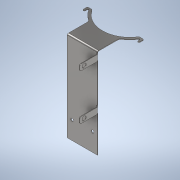
# Autodesk Inventor part: Glass fixer plate
Saved by Autodesk Inventor 2020.3 (Build 243373000, 373)
## iProperties
Created: 2020-06-30
Part Number: Glass fixer plate
Material: Steel, Carbon
Document SubType Name: Sheet Metal
Designer: Bruno
Density: 7.85 g/cm^3
Sheet Metal Rule: Default_mm
Appearance: Semi-Polished
Author: Bruno
Autodesk Inventor part; units mm, degrees
ref_plane "YZ Plane" through (0, 0, 0) normal (1, 0, 0) x (0, 1, 0)
ref_plane "XZ Plane" through (0, 0, 0) normal (0, 1, 0) x (-1, 0, 0)
ref_plane "XY Plane" through (0, 0, 0) normal (0, 0, 1) x (1, 0, 0)
sketch "Sketch1" plane through (0, 0, 0) normal (0, 0, 1) x (1, 0, 0)
  line L0 (0, 0) -> (50, 0)
  line L1 (50, 0) -> (50, 150)
  line L2 (50, 150) -> (0, 150)
  line L3 (0, 150) -> (0, 0)
  dimension "d0" = 50
  dimension "d1" = 150
  measures "d0" distance of L2.end L1.end
  measures "d1" distance of L1.end L0.end
extrude "Plate1" add sketch "Sketch1" along normal blind 1
sketch "Sketch2" plane through (50, 149, 1) normal (0, 1, 0) x (-1, 0, 0)
  line L0 (50, 0) -> (0, 0)
  line L1 (0, 0) -> (0, -79)
  line L2 (0, -79) -> (50, -79)
  line L3 (50, -79) -> (50, 0)
  constraints: 6 end point, 1 horizontal, 1 perpendicular, 1 vertical
edge flange "Flange1" height 79 angle 90 thickness 1 bend radius 1 thickness toward (0, 1, 0) relief straight relief width 1 relief depth 0.5 edges at (25, 150, 0) wall of the first edge with corners at (0, 149, 1) (50, 149, 1) (50, 149, -78) (0, 149, -78)
bend "Bend1"
corner "Corner1"
sketch "Sketch4" plane through (0, 150, -78) normal (0, 1, 0) x (1, 0, 0)
  line L0 (0, 0) -> (50, 0)
  line L1 (0, 0) -> (-40, 0)
  line L2 (-40, 0) -> (-40, -40)
  line L3 (-40, -40) -> (0, -40)
  line L4 (0, -40) -> (0, 0)
  line L5 (50, -77) -> (50, 0)
  line L6 (50, 0) -> (90, 0)
  line L7 (90, 0) -> (90, -40)
  line L8 (90, -40) -> (50, -40)
  line L9 (50, -40) -> (50, 0)
  point P0 (0, -78)
  dimension "d14" = 40
  dimension "d15" = 40
  dimension "d16" = 40
  dimension "d17" = 40
  measures "d14" distance of L3.end L2.end
  measures "d15" distance of L2.end L1.end
  measures "d16" distance of L7.end L8.end
  measures "d17" distance of L6.end L7.end
sheet face with bend "Face2" sketch "Sketch4" thickness 1 toward (0, -1, 0) bend radius 1 relief straight relief width 1 relief depth 0.5
bend "Bend2"
fillet "Corner Round7" radius 6 2 edges at (0, 149.5, -38) (50, 149.5, -38)
sketch "Sketch3" plane through (0, 150, -78) normal (0, 1, 0) x (1, 0, 0)
  line L0 (0, 0) -> (50, 0) projected
  circle A0 centre (25, 0) radius 45.5
  arc A1 (-16.7744, -26.5) -> (66.7744, -26.5) centre (25, 0) ccw
  arc A2 (0, -46) -> (-6, -40) centre (-6, -46) ccw projected
  circle A3 centre (-6, -46) radius 6
  arc A4 (56, -40) -> (50, -46) centre (56, -46) ccw projected
  circle A5 centre (56, -46) radius 6
  line L1 (-40, -40) -> (-6, -40) projected
  line L2 (-6, -40) -> (-40, -40)
  line L3 (-40, 0) -> (-40, -40) projected
  line L4 (-40, -40) -> (-40, 0)
  line L5 (-40, 0) -> (-20.5, 0)
  line L6 (90, 0) -> (-40, 0) projected
  line L7 (56, -40) -> (90, -40) projected
  line L8 (56, -40) -> (90, -40)
  line L9 (90, -40) -> (90, 0) projected
  line L10 (90, -40) -> (90, 0)
  line L11 (90, 0) -> (70.5, 0)
  line L12 (25, 0) -> (25, -45.5)
  line L13 (25, -45.5) -> (25, -23.5) construction
  line L14 (25, -23.5) -> (63.9615, -23.5) construction
  line L15 (63.9615, -23.5) -> (69.9615, -23.5)
  line L16 (63.9615, -23.5) -> (69.9615, -23.5) construction
  line L17 (71.9615, -25.5) -> (71.9615, -30)
  line L18 (70.4615, -31.5) -> (70.4615, -31.5)
  line L19 (25, -23.5) -> (-13.9615, -23.5) construction
  line L20 (-13.9615, -23.5) -> (-19.9615, -23.5)
  line L21 (-13.9615, -23.5) -> (-7.9615, -23.5) construction
  line L22 (-21.9615, -25.5) -> (-21.9615, -30)
  line L23 (-20.4615, -31.5) -> (-20.4615, -31.5)
  arc A6 (-16.7744, -26.5) -> (66.7744, -26.5) centre (25, 0) ccw
  line L24 (-18.9615, -30) -> (-18.9615, -27.5)
  line L25 (-17.9615, -26.5) -> (-16.7744, -26.5)
  line L26 (68.9615, -30) -> (68.9615, -27.5)
  line L27 (67.9615, -26.5) -> (66.7744, -26.5)
  arc A7 (-19.9615, -23.5) -> (-21.9615, -25.5) centre (-19.9615, -25.5) ccw
  arc A8 (-21.9615, -30) -> (-20.4615, -31.5) centre (-20.4615, -30) ccw
  arc A9 (-20.4615, -31.5) -> (-18.9615, -30) centre (-20.4615, -30) ccw
  arc A10 (-17.9615, -26.5) -> (-18.9615, -27.5) centre (-17.9615, -27.5) ccw
  arc A11 (71.9615, -25.5) -> (69.9615, -23.5) centre (69.9615, -25.5) ccw
  arc A12 (70.4615, -31.5) -> (71.9615, -30) centre (70.4615, -30) ccw
  arc A13 (68.9615, -30) -> (70.4615, -31.5) centre (70.4615, -30) ccw
  arc A14 (68.9615, -27.5) -> (67.9615, -26.5) centre (67.9615, -27.5) ccw
  point P0 (0, -78)
  point P1 (52.6469, -41.0244)
  point P2 (-2.6469, -41.0244)
  point P3 (71.9615, -23.5)
  point P4 (71.9615, -31.5)
  point P5 (68.9615, -31.5)
  point P6 (-21.9615, -23.5)
  point P7 (-21.9615, -31.5)
  point P8 (-18.9615, -31.5)
  point P9 (-18.9615, -26.5)
  point P10 (68.9615, -26.5)
  point P11 (-2.6469, -41.0244)
  point P12 (52.6469, -41.0244)
  point P13 (70.4615, -31.5)
  dimension "d13" = 91
  dimension "d84" = 22
  dimension "d85" = 8
  dimension "d86" = 0
  dimension "d87" = 8
  dimension "d88" = 3
  dimension "d89" = 8
  dimension "d90" = 180
  dimension "d91" = 8
  dimension "d92" = 90
  dimension "d93" = 3
  dimension "d95" = 5
  dimension "d96" = 5
  dimension "d97" = 2
  dimension "d98" = 1.5
  dimension "d99" = 1.5
  dimension "d100" = 1
  dimension "d101" = 2
  dimension "d102" = 1.5
  dimension "d103" = 1
  constraints: 44 end point, 25 point on circle, 19 point on line, 18 tangent, 13 centre point, 7 perpendicular, 6 collinear, 5 horizontal, 4 coincident, 3 vertical, 1 concentric, 1 midpoint
  measures "d13" diameter of A0
  measures "d84" distance of L12.end L13.end
  measures "d85" distance of L14.end point (71.962, -23.5)
  measures "d86" distance between parallel lines of L15 L16
  measures "d87" distance of point (71.962, -23.5) point (71.962, -31.5)
  measures "d88" distance of point (71.962, -31.5) point (68.962, -31.5)
  measures "d89" distance of L19.end point (-21.962, -23.5)
  measures "d90" angle of L20 L21
  measures "d91" distance of point (-21.962, -23.5) point (-21.962, -31.5)
  measures "d92" angle of L22 L20
  measures "d93" distance of point (-21.962, -31.5) point (-18.962, -31.5)
  measures "d95" distance of point (-18.962, -31.5) point (-18.962, -26.5)
  measures "d96" distance of point (68.962, -31.5) point (68.962, -26.5)
  measures "d97" radius of A7
  measures "d98" radius of A8
  measures "d99" radius of A9
  measures "d100" radius of A10
  measures "d101" radius of A11
  measures "d102" radius of A12
  measures "d103" radius of A14
extrude "Extrusion1" cut sketch "Sketch3" against normal through all contours L6 A0 L0 | L0 L12 A0 L6 | L0 L6 A0 L12 | A0 L20 A7 L22 A8 A9 L24 A10 L25 A1 A2 L1 L3 L5 | L6 L9 L7 A4 A1 L27 A14 L26 A13 A12 L17 A11 L15 A0
sketch "Sketch5" plane through (0, 150, -1) normal (0, 1, 0) x (1, 0, 0)
  arc A0 (-13.9615, 53.5) -> (63.9615, 53.5) centre (25, 77) ccw projected
  point P0 (0, -1)
  point P1 (70.5, 77)
  point P2 (-20.5, 77)
sketch "Sketch7" plane through (0, 0, 1) normal (0, 0, 1) x (1, 0, 0)
  line L0 (50, 0) -> (0, 0) projected
  line L1 (0, 0) -> (0, 148) projected
  line L2 (50, 148) -> (50, 0) projected
  point P0 (8, 30)
  point P1 (42, 30)
  dimension "d37" = 30
  dimension "d38" = 8
  dimension "d39" = 8
  constraints: 1 horizontal alignment
  measures "d37" distance from line of L0 point (8, 30)
  measures "d38" distance from line of L1 point (8, 30)
  measures "d39" distance from line of L2 point (42, 30)
hole "Hole1" at (8, 30, 1) at (42, 30, 1) direction (0, 0, -1) diameter 4.5 end through all
fillet "Corner Round12" radius 1 1 edges at (-16.7744, 149.5, -51.5)
fillet "Corner Round13" radius 1 1 edges at (66.7744, 149.5, -51.5)
fillet "Corner Round14" radius 3 1 edges at (63.9615, 149.5, -54.5)
fillet "Corner Round15" radius 3 1 edges at (-13.9615, 149.5, -54.5)
sketch "Sketch10" plane through (0, 150, -1) normal (0, 1, 0) x (1, 0, 0)
  arc A0 (70.7921, 70.1608) -> (-20.7921, 70.1608) centre (25, 77) ccw
  line L0 (25, 77) -> (25, 30.7) construction
  line L1 (-17.3207, 50.5) -> (-17.9615, 50.5) projected
  line L2 (-18.9615, 47) -> (-18.9615, 49.5) projected
  line L3 (-17.6615, 49.2) -> (-20.7921, 70.1608)
  line L4 (-20.7921, 70.1608) -> (25, 70.1608) construction
  line L5 (68.9615, 49.5) -> (68.9615, 47) projected
  line L6 (67.3207, 50.5) -> (67.9615, 50.5) projected
  line L7 (67.6615, 49.2) -> (70.7921, 70.1608)
  line L8 (70.7921, 70.1608) -> (25, 70.1608) construction
  point P0 (0, -1)
  dimension "d109" = 92.6
  dimension "d115" = 1.3
  dimension "d116" = 1.3
  dimension "d117" = 45.7921
  dimension "d118" = 6.8392
  dimension "d119" = 1.3
  dimension "d120" = 1.3
  dimension "d121" = 45.7921
  constraints: 10 end point, 2 point on circle, 2 tangent, 1 centre point, 1 coincident, 1 perpendicular, 1 point on line, 1 vertical
  measures "d109" diameter of A0
  measures "d115" distance from line of L2 L3.start
  measures "d116" distance from line of L1 L3.start
  measures "d117" distance of L3.end L4.end
  measures "d118" distance from line of point (25, 77) L4
  measures "d119" distance from line of L5 L7.start
  measures "d120" distance from line of L7.start L6
  measures "d121" distance of L7.end L4.end
sketch "Sketch13" plane through (50, 0, 0) normal (1, 0, 0) x (0, 0, -1)
  line L0 (-1, 0) -> (-1, 148)
  line L1 (-1, 146) -> (-31, 146)
  line L2 (-31, 146) -> (-31, 136)
  line L3 (-31, 136) -> (-1, 136)
  line L4 (-1, 136) -> (-1, 146)
  line L5 (-1, 70) -> (-31, 70)
  line L6 (-31, 70) -> (-31, 60)
  line L7 (-31, 60) -> (-1, 60)
  line L8 (-1, 60) -> (-1, 70)
  point P0 (0, 0)
  dimension "d133" = 30
  dimension "d134" = 10
  dimension "d135" = 146
  dimension "d136" = 30
  dimension "d137" = 10
  dimension "d138" = 66
  measures "d133" distance of L3.end L2.end
  measures "d134" distance of L2.end L1.end
  measures "d135" distance from line of L0.start L1
  measures "d136" distance of L7.end L6.end
  measures "d137" distance of L6.end L5.end
  measures "d138" distance between parallel lines of L5 L3
sheet face with bend "Face4" sketch "Sketch13" thickness 1 toward (1, 0, 0) bend radius 1 relief straight relief width 1 relief depth 0.5
bend "Bend4"
sketch "Sketch14" plane through (50, 0, 0) normal (-1, 0, 0) x (0, 0, 1)
  line L0 (1, 0) -> (1, 148) projected
  line L1 (2, 146) -> (31, 146) projected
  line L2 (2, 70) -> (31, 70) projected
  point P0 (0, 0)
  point P1 (24, 141)
  point P2 (24, 65)
  dimension "d144" = 23
  dimension "d145" = 5
  dimension "d146" = 5
  dimension "d154" = 76
  constraints: 1 vertical alignment
  measures "d144" distance from line of L0 point (24, 141)
  measures "d145" distance from line of L1 point (24, 141)
  measures "d146" distance from line of point (24, 65) L2
  measures "d154" distance of point (24, 65) point (24, 141)
hole "Hole2" at (50, 141, 24) at (50, 65, 24) direction (1, 0, 0) diameter 7 end through all
fillet "Fillet1" radius 2 4 edges at (50.5, 146, 31) (50.5, 136, 31) (50.5, 70, 31) (50.5, 60, 31)
equation "\"d39\" = d38"
equation "\"d145\" = 0.5 * d134"
equation "\"d146\" = d145"
equation "\"d16\" = d14"
equation "\"d17\" = d15"
equation "\"d45\" = Thickness"
equation "\"d137\" = d134"
equation "\"d152\" = Thickness"
equation "\"d2\" = Thickness"
equation "\"d3\" = BendReliefWidth"
equation "\"d4\" = BendReliefDepth"
equation "\"d5\" = MinimumRemnant"
equation "\"d6\" = TransitionRadius"
equation "\"d9\" = BendRadius"
equation "\"d10\" = CornerReliefSize"
equation "\"d11\" = GapSize"
equation "\"d12\" = JacobiRadiusSize"
equation "\"d18\" = BendRadius"
equation "\"d19\" = BendReliefWidth"
equation "\"d21\" = MinimumRemnant"
equation "\"d20\" = BendReliefDepth"
equation "\"d22\" = TransitionRadius"
equation "\"d139\" = BendRadius"
equation "\"d140\" = BendReliefWidth"
equation "\"d142\" = MinimumRemnant"
equation "\"d141\" = BendReliefDepth"
equation "\"d143\" = TransitionRadius"
equation "\"BendRadius\" = Thickness"
equation "\"BendReliefWidth\" = Thickness"
equation "\"BendReliefDepth\" = 0.5 * Thickness"
equation "\"CornerReliefSize\" = 4 * Thickness"
equation "\"MinimumRemnant\" = 2 * Thickness"
equation "\"TransitionRadius\" = BendRadius"
equation "\"JacobiRadiusSize\" = BendRadius"
equation "\"GapSize\" = Thickness"
equation "\"Thickness\" = 1"
body "Solid1"
